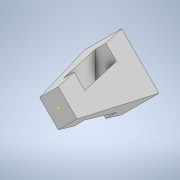
# Autodesk Inventor part: Деталь1
Saved by Autodesk Inventor 2020 (Build 240168000, 168)
## iProperties
Created: 2020-03-16
Part Number: Деталь1
Material: Типовые
Document SubType Name: Modeling
Designer: Trickster2038
Density: 1 g/cm^3
Appearance: По умолчанию
Author: Trickster2038
Autodesk Inventor part; units mm, degrees
ref_plane "YZ Plane" through (0, 0, 0) normal (1, 0, 0) x (0, 1, 0)
sketch "Эскиз1" plane through (0, 0, 0) normal (0, 0, 1) x (1, 0, 0)
  line L0 (-35.3564, 0.0006) -> (-0.0011, 35.3559)
  line L1 (-35.3564, 0.0006) -> (-0.0011, -35.3548)
  line L2 (-0.0011, -35.3548) -> (35.3543, 0.0006)
  line L3 (35.3543, 0.0006) -> (-0.0011, 35.3559)
  point P0 (0, 0)
  point P1 (0, 0)
  constraints: 8 end point, 1 coincident, 1 perpendicular
sketch "Эскиз2" plane through (0, 0, 0) normal (0, 0, 1) x (1, 0, 0)
  point P0 (0, 0)
ref_plane "РабПлоскость1" through (0, 0, 60) normal (0, 0, 1) x (1, 0, 0)
sketch "Эскиз3" plane through (0, 0, 60) normal (0, 0, 1) x (1, 0, 0)
  line L0 (-17.6777, 0) -> (0, 17.6777)
  line L1 (0, 17.6777) -> (17.6777, 0)
  line L2 (17.6777, 0) -> (0, -17.6777)
  line L3 (0, -17.6777) -> (-17.6777, 0)
  point P0 (0, 0)
  constraints: 8 end point, 2 perpendicular
sketch "Эскиз4" plane through (0, 0, 60) normal (0, 0, 1) x (1, 0, 0)
  point P0 (0, 0)
sketch "Эскиз5" plane through (0, 0, 60) normal (0, 0, 1) x (1, 0, 0)
  point P0 (0, 0)
sketch "Эскиз6" plane through (0, 0, 0) normal (0, 0, 1) x (1, 0, 0)
  point P0 (0, 0)
sketch "Эскиз7" plane through (0, 0, 0) normal (0, 0, 1) x (1, 0, 0)
  point P0 (0, 0)
loft "Лофт1" add profiles "Эскиз1", "Эскиз3"
sketch "Эскиз8" plane through (0, 0, 0) normal (0, 1, 0) x (-1, 0, 0)
  point P0 (0, 0)
ref_plane "РабПлоскость2" through (0, 70, 0) normal (0, 1, 0) x (-1, 0, 0)
sketch "Эскиз9" plane through (0, 70, 0) normal (0, 1, 0) x (-1, 0, 0)
  line L0 (-9.9989, 45) -> (10.0011, 45)
  line L1 (10.0011, 45) -> (10.0011, 15)
  line L2 (10.0011, 15) -> (-9.9989, 15)
  line L3 (-9.9989, 15) -> (-9.9989, 45)
  line L4 (0.0011, 0) -> (-35.3543, 0) projected
  point P0 (0, 0)
  constraints: 8 end point, 2 parallel, 1 horizontal, 1 perpendicular
extrude "Выдавливание1" cut sketch "Эскиз9" against normal blind 110
